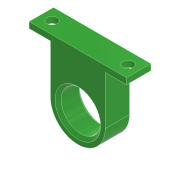
# Autodesk Inventor part: driver gear stopper
Saved by Autodesk Inventor 2022 (Build 260153000, 153)
## iProperties
Created: 2024-07-09
Part Number: driver gear stopper
Material: Generic
Document SubType Name: Modeling
Designer: david
Density: 1 g/cm^3
Appearance: Smooth - Dark Forest Green
Author: david
Autodesk Inventor part; units mm, degrees
ref_plane "YZ Plane" through (0, 0, 0) normal (1, 0, 0) x (0, 1, 0)
ref_plane "XZ Plane" through (0, 0, 0) normal (0, 1, 0) x (-1, 0, 0)
ref_plane "XY Plane" through (0, 0, 0) normal (0, 0, 1) x (1, 0, 0)
sketch "Sketch2" plane through (0, 0, 0) normal (0, 0, 1) x (1, 0, 0)
  line L0 (0, 0) -> (0, -18) construction
  line L1 (-9, 0) -> (-9, -18)
  line L2 (9, -18) -> (9, 0)
  arc A0 (9, 0) -> (-9, 0) centre (0, 0) ccw construction
  arc A1 (-9, -18) -> (9, -18) centre (0, -18) ccw
  arc A2 (6.5, -18) -> (-6.5, -18) centre (0, -18) ccw
  circle A3 centre (0, -18) radius 5 construction
  line L3 (-9, 0) -> (9, 0)
  line L4 (9, -18) -> (6.5, -18)
  arc A4 (-6.5, -18) -> (0, -24.5) centre (0, -18) ccw
  arc A5 (0, -24.5) -> (6.5, -18) centre (0, -18) ccw
  line L5 (-6.5, -18) -> (-9, -18)
  line L6 (6.5, -18) -> (-6.5, -18) construction
  line L7 (9, -18) -> (6.5, -18)
  line L8 (-9, -18) -> (-6.5, -18)
  point P0 (0, -9)
  dimension "d2" = 2.5
  dimension "d3" = 10
  dimension "d4" = 1.5
  dimension "d5" = 18
  constraints: 20 end point, 10 point on circle, 6 centre point, 4 perpendicular, 4 tangent, 2 coincident, 2 horizontal, 1 midpoint, 1 parallel, 1 point on line, 1 vertical
  measures "d2" distance edge to line of A2 L2
  measures "d3" diameter of A3
  measures "d4" radial gap between concentric circles of A2 A3
  measures "d5" distance of L0.start L0.end
extrude "Extrusion1" add sketch "Sketch2" along normal mid plane 8 contours L3 L2 L4 A2 L5 L1 | L5 A4 A5 L4 A1
sketch "Sketch3" plane through (-9, 0, 4) normal (0, 1, 0) x (1, 0, 0)
  line L0 (-7, 0) -> (25, 0)
  line L1 (25, 0) -> (25, 8)
  line L2 (25, 8) -> (-7, 8)
  line L3 (-7, 8) -> (-7, 0)
  line L4 (-7, 0) -> (25, 8) construction
  line L5 (25, 0) -> (-7, 8) construction
  line L6 (0, 8) -> (18, 8) projected
  line L7 (0, 8) -> (0, 0) projected
  point P0 (9, 4)
  dimension "d8" = 7
  constraints: 12 end point, 2 midpoint, 2 parallel, 1 collinear, 1 horizontal, 1 perpendicular
  measures "d8" distance between parallel lines of L7 L3
extrude "Extrusion2" add sketch "Sketch3" against normal blind 2
sketch "Sketch4" plane through (-9, -2, 4) normal (0, -1, 0) x (1, 0, 0)
  line L0 (18, -8) -> (0, -8) construction
  line L1 (-7, 0) -> (0, 0) construction
  line L2 (-7, -8) -> (-7, 0) construction
  line L3 (0, 0) -> (18, 0) construction
  line L4 (25, 0) -> (25, -8) construction
  line L5 (25, -8) -> (18, -8) construction
  line L6 (0, -8) -> (0, 0) construction
  line L7 (0, -8) -> (-7, -8) construction
  line L8 (18, 0) -> (25, 0) construction
  line L9 (18, 0) -> (18, -8) construction
  line L10 (0, 0) -> (0, -8) projected
  line L11 (0, 0) -> (-7, 0) projected
  line L12 (-7, 0) -> (-7, -8) projected
  line L13 (-7, -8) -> (0, -8) projected
  line L14 (18, -8) -> (18, 0) projected
  line L15 (18, -8) -> (25, -8) projected
  line L16 (25, -8) -> (25, 0) projected
  line L17 (25, 0) -> (18, 0) projected
  point P0 (-3.5, -4)
  point P1 (21.5, -4)
  point P2 (21.5, 0)
  point P3 (-3.5, 0)
  point P4 (25, -4)
  point P5 (25, -4)
  constraints: 4 midpoint, 2 horizontal alignment, 2 vertical alignment
hole "Hole1" at (-12.5, -2, 0) at (12.5, -2, 0) direction (0, 1, 0) diameter 3.4 end through all
chamfer "Chamfer2" distance 1 angle 45 2 edges at (0, -11.5, -4) (0, -11.5, 4)
body "Solid1"
